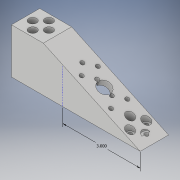
# Autodesk Inventor part: IntakeCchannelMount
Saved by Autodesk Inventor 2018 (Build 220112000, 112)
## iProperties
Created: 2018-01-30
Part Number: IntakeCchannelMount
Material: Generic
Document SubType Name: Modeling
Designer: 1452927
Density: 1 g/cm^3
Appearance: Default
Author: 1452927
Autodesk Inventor part; units mm, degrees
ref_plane "YZ Plane" through (0, 0, 0) normal (1, 0, 0) x (0, 1, 0)
sketch "Sketch17" plane through (0, 0, 0) normal (0, 0, 1) x (1, 0, 0)
  line L0 (0, 0) -> (127, 0)
  line L1 (127, 0) -> (31.3739, 44.5912)
  line L2 (0, 44.5912) -> (0, 0)
  line L3 (0, 44.5912) -> (31.3739, 44.5912)
  dimension "d78" = 127
  dimension "d79" = 25
  constraints: 8 end point, 2 horizontal, 1 perpendicular
  measures "d78" distance of L0.start L0.end
  measures "d79" angle of L0 L1
extrude "Extrusion20" add sketch "Sketch17" along normal blind 25.4
sketch "Sketch18" plane through (0, 0, 0) normal (0, -1, 0) x (1, 0, 0)
  line L0 (127.0002, 25.3999) -> (0.1269, 25.3999)
  line L1 (0.1269, 25.3999) -> (0.1269, -0.0001)
  line L2 (127.0002, -0.0001) -> (0.1269, -0.0001)
  line L3 (127.0002, 25.3999) -> (127.0002, -0.0001)
  circle A0 centre (111.0002, 22) radius 1.85 projected
  circle A1 centre (111.0002, 6) radius 1.85 projected
  circle A2 centre (119.0002, 14) radius 1.85 projected
  circle A3 centre (103.0002, 14) radius 1.85 projected
  circle A4 centre (7.0002, 14) radius 1.85 projected
  circle A5 centre (15.0002, 22) radius 1.85 projected
  circle A6 centre (15.0002, 6) radius 1.85 projected
  circle A7 centre (23.0002, 14) radius 1.85 projected
  point P0 (0, 0)
  point P1 (50.8002, 25.3999)
  constraints: 8 end point
sketch "Sketch19" plane through (0, 0, 25.4) normal (0, 0, 1) x (1, 0, 0)
  line L0 (0, 0) -> (127, 0) projected
  line L1 (127, 0) -> (31.3739, 44.5912) projected
  line L2 (31.3739, 44.5912) -> (0, 44.5912) projected
  line L3 (0, 44.5912) -> (0, 0) projected
extrude "Extrusion21" add sketch "Sketch19" along normal blind 2.54
extrude "Extrusion22" cut sketch "Sketch18" against normal up to next contours A0 | A1 | A2 | A3 | A4 | A5 | A6 | A7
ref_plane "Work Plane11" through (0, 3.81, 0) normal (0, -1, 0) x (1, 0, 0)
sketch "Sketch20" plane through (0, 3.81, 0) normal (0, -1, 0) x (1, 0, 0)
  circle A0 centre (15.0002, 22) radius 1.85 projected
  circle A1 centre (15.0002, 22) radius 3.9751
  circle A2 centre (7.0002, 14) radius 1.85 projected
  circle A3 centre (7.0002, 14) radius 3.9751
  circle A4 centre (15.0002, 6) radius 1.85 projected
  circle A5 centre (15.0002, 6) radius 3.9751
  circle A6 centre (23.0002, 14) radius 1.85 projected
  circle A7 centre (23.0002, 14) radius 3.9751
  circle A8 centre (103.0002, 14) radius 1.85 projected
  circle A9 centre (103.0002, 14) radius 3.9751
  circle A10 centre (111.0002, 22) radius 1.85 projected
  circle A11 centre (111.0002, 22) radius 3.9751
  circle A12 centre (111.0002, 6) radius 1.85 projected
  circle A13 centre (111.0002, 6) radius 3.9751
  circle A14 centre (119.0002, 14) radius 1.85 projected
  circle A15 centre (119.0002, 14) radius 3.9751
  point P0 (0, 0)
  dimension "d100" = 7.9502
  dimension "d101" = 7.9502
  dimension "d102" = 7.9502
  dimension "d103" = 7.9502
  dimension "d104" = 7.9502
  dimension "d105" = 7.9502
  dimension "d106" = 7.9502
  dimension "d107" = 7.9502
  constraints: 8 centre point, 8 coincident
  measures "d100" diameter of A1
  measures "d101" diameter of A7
  measures "d102" diameter of A5
  measures "d103" diameter of A3
  measures "d104" diameter of A9
  measures "d105" diameter of A11
  measures "d106" diameter of A13
  measures "d107" diameter of A15
extrude "Extrusion23" cut sketch "Sketch20" against normal up to next
ref_plane "Work Plane12" through (28.6903, 38.8361, 27.94) normal (0.4226, 0.9063, 0) x (0.9063, -0.4226, 0)
sketch "Sketch21" plane through (0, 0, 0) normal (0, -1, 0) x (1, 0, 0)
  line L0 (30.6202, 24.13) -> (95.3802, 24.13)
  line L1 (95.3802, 24.13) -> (95.3802, 0)
  line L2 (95.3802, 0) -> (30.6202, 0)
  line L3 (30.6202, 0) -> (30.6202, 24.13)
  line L4 (0, 27.94) -> (127, 27.94) construction
  line L5 (0, 0) -> (127, 0) construction
  circle A0 centre (23.0002, 14) radius 1.85 construction
  circle A1 centre (103.0002, 14) radius 1.85 construction
  dimension "d112" = 3.81
  dimension "d113" = 0
  dimension "d114" = 7.62
  dimension "d115" = 7.62
  constraints: 8 end point, 2 parallel, 1 horizontal, 1 perpendicular
  measures "d112" distance between parallel lines of L4 L0
  measures "d113" distance between parallel lines of L5 L2
  measures "d114" distance from line of L3 A0.centre
  measures "d115" distance from line of A1.centre L1
extrude "Extrusion24" cut sketch "Sketch21" against normal up to surface surface through (28.6903, 38.8361, 27.94) normal (0.4226, 0.9063, 0)
sketch "Sketch23" plane through (0, 0, 27.94) normal (0, 0, 1) x (1, 0, 0)
  line L0 (0, 0) -> (127, 0) construction
  line L1 (127, 0) -> (50.8, 0) construction
  line L2 (50.8, 0) -> (50.8, 35.5326) construction
  line L3 (127, 0) -> (31.3739, 44.5912) construction
  dimension "d119" = 76.2
  constraints: 4 end point, 2 point on line, 1 perpendicular
  measures "d119" distance of L0.end L1.end
sketch "Sketch24" plane through (31.3739, 44.5912, 27.94) normal (0.4226, 0.9063, 0) x (0.9063, -0.4226, 0)
  circle A0 centre (35.1489, 5.94) radius 1.85 projected
  circle A1 centre (27.1489, 13.94) radius 1.85 projected
  circle A2 centre (35.1489, 21.94) radius 1.85 projected
  circle A3 centre (43.1489, 13.94) radius 1.85 projected
  circle A4 centre (51.1489, 13.94) radius 4 projected
  circle A5 centre (59.1489, 13.94) radius 1.85 projected
  circle A6 centre (67.1489, 5.94) radius 1.85 projected
  circle A7 centre (75.1489, 13.94) radius 1.85 projected
  circle A8 centre (67.1489, 21.94) radius 1.85 projected
  circle A9 centre (51.1489, 13.94) radius 6.35
  circle A10 centre (67.1489, 5.94) radius 1.9542
  circle A11 centre (75.1489, 13.94) radius 3.9195
  circle A12 centre (67.1489, 21.94) radius 1.9542
  circle A13 centre (59.1489, 13.94) radius 1.9542
  circle A14 centre (43.1489, 13.94) radius 1.9542
  circle A15 centre (35.1489, 5.94) radius 1.9542
  circle A16 centre (27.1489, 13.94) radius 1.9542
  circle A17 centre (35.1489, 21.94) radius 1.9542
  point P0 (-9.5894, 27.94)
  dimension "d120" = 12.7
  dimension "d125" = 3.9084
  dimension "d126" = 3.9084
  dimension "d127" = 3.9084
  dimension "d128" = 3.9084
  dimension "d129" = 3.9084
  dimension "d130" = 3.9084
  dimension "d131" = 3.9084
  constraints: 9 centre point, 9 coincident
  measures "d120" diameter of A9
  measures "d125" diameter of A14
  measures "d126" diameter of A15
  measures "d127" diameter of A16
  measures "d128" diameter of A17
  measures "d129" diameter of A13
  measures "d130" diameter of A10
  measures "d131" diameter of A12
extrude "Extrusion25" cut sketch "Sketch24" against normal up to surface (6.35 mm away) contours A0 | A1 | A2 | A3 A9 | A3 A9 A14 | A9 A3 | A3 A9 A14 | A9 A13 A14 | A13 A9 A5 | A9 A5 A13 | A9 A5 | A5 A9 | A4 | A6 | A8 | A10 | A12 | A15 | A16 | A17
sketch "Sketch27" plane through (95.3802, 0, 24.13) normal (0, 0, -1) x (-1, 0, 0)
  line L0 (64.76, 0) -> (0, 0) projected
  line L1 (64.76, 0) -> (64.76, 37.7416)
  line L2 (64.76, 37.7416) -> (47.4149, 29.6534)
  line L3 (43.8558, 28.1884) -> (40.3136, 26.5366) projected
  line L4 (47.4149, 29.6534) -> (61.2425, 0)
  line L5 (61.2425, 0) -> (64.76, 0)
  point P0 (95.3802, 0)
  constraints: 8 end point, 2 perpendicular, 1 parallel, 1 vertical
extrude "Extrusion27" add sketch "Sketch27" along normal up to surface (24.13 mm away)
body "Solid2"
